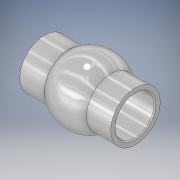
# Autodesk Inventor part: Bola_libertad_grande
Saved by Autodesk Inventor 2019 (Build 230136000, 136)
## iProperties
Created: 2019-09-23
Part Number: Bola_libertad_grande
Material: Genérico
Document SubType Name: Modeling
Designer: axelj
Density: 1 g/cm^3
Appearance: Aluminio - Pulido
Author: axelj
Autodesk Inventor part; units mm, degrees
ref_plane "XZ Plane" through (0, 0, 0) normal (0, 1, 0) x (-1, 0, 0)
ref_plane "XY Plane" through (0, 0, 0) normal (0, 0, 1) x (1, 0, 0)
sketch "Boceto1" plane through (0, 0, 0) normal (0, 1, 0) x (-1, 0, 0)
  arc A0 (-2.5, 0) -> (2.5, 0) centre (0, 0) ccw
  line L0 (-2.5, 0) -> (2.5, 0)
  dimension "d0" = 5
  constraints: 2 end point, 2 point on circle, 1 centre point, 1 coincident, 1 horizontal
  measures "d0" diameter of A0
revolve "Revolución1" add sketch "Boceto1" angle 360 about axis through (2.5, 0, 0) along (-1, 0, 0)
ref_plane "Plano de trabajo1" through (2.5, 0, 0) normal (1, 0, 0) x (0, 1, 0)
sketch "Boceto2" plane through (2.5, 0, 0) normal (1, 0, 0) x (0, 1, 0)
  circle A0 centre (0, 0) radius 1.5
  circle A1 centre (0, 0) radius 1.9
  dimension "d3" = 3
  dimension "d4" = 3.8
  constraints: 2 centre point, 2 coincident
  measures "d3" diameter of A0
  measures "d4" diameter of A1
extrude "Extrusión1" add sketch "Boceto2" along normal blind 1 and the other way blind 6
sketch "Boceto3" plane through (2.5, 0, 0) normal (1, 0, 0) x (0, 1, 0)
  circle A0 centre (0, 0) radius 1.5
  constraints: 1 centre point, 1 coincident
extrude "Extrusión2" cut sketch "Boceto3" against normal blind 10000
fillet "Empalme1" radius 0.08 2 edges at (-3.5, -1.5, 0) (3.5, -1.5, 0)
